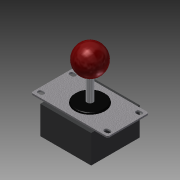
# Autodesk Inventor part: Sanwa_Joystick_JLF-TP-8YT
Saved by Autodesk Inventor 2013 (Build 170138000, 138)
## iProperties
Created: 2012-06-19
Part Number: Sanwa_Joystick_JLF-TP-8YT
Material: Generic
Document SubType Name: Sheet Metal
Designer: bbooth
Density: 1 g/cm^3
Sheet Metal Rule: Default
Author: bbooth
Autodesk Inventor part; units mm, degrees
ref_plane "YZ Plane" through (0, 0, 0) normal (1, 0, 0) x (0, 1, 0)
ref_plane "XZ Plane" through (0, 0, 0) normal (0, 1, 0) x (-1, 0, 0)
ref_plane "XY Plane" through (0, 0, 0) normal (0, 0, 1) x (1, 0, 0)
sketch "Sketch2" plane through (0, 0, 0) normal (0, 1, 0) x (-1, 0, 0)
  line L0 (-49, 26.5) -> (49, 26.5)
  line L1 (49, 26.5) -> (49, -26.5)
  line L2 (49, -26.5) -> (-49, -26.5)
  line L3 (-49, -26.5) -> (-49, 26.5)
  point P0 (0, 0)
  point P1 (0, -26.5)
  point P2 (49, 0)
  dimension "d5" = 98
  dimension "d7" = 53
  constraints: 8 end point, 2 midpoint, 2 parallel, 1 horizontal, 1 horizontal alignment, 1 perpendicular, 1 vertical alignment
  measures "d5" distance of L2.end L1.end
  measures "d7" distance between parallel lines of L0 L2
extrude "Extrusion1" add sketch "Sketch2" along normal blind 2
sketch "Sketch3" plane through (0, 2, 0) normal (0, 1, 0) x (1, 0, 0)
  line L0 (-49, -26.5) -> (49, -26.5) projected
  line L1 (49, -26.5) -> (49, 26.5) projected
  line L2 (49, 26.5) -> (-49, 26.5) projected
  line L3 (-49, 26.5) -> (-49, -26.5) projected
  arc A0 (43.75, 17.5) -> (43.75, 23) centre (43.75, 20.25) ccw
  arc A1 (41.25, 23) -> (41.25, 17.5) centre (41.25, 20.25) ccw
  line L4 (41.25, 23) -> (43.75, 23)
  line L5 (41.25, 17.5) -> (43.75, 17.5)
  arc A2 (-41.25, 17.5) -> (-41.25, 23) centre (-41.25, 20.25) ccw
  arc A3 (-43.75, 23) -> (-43.75, 17.5) centre (-43.75, 20.25) ccw
  line L6 (-43.75, 23) -> (-41.25, 23)
  line L7 (-43.75, 17.5) -> (-41.25, 17.5)
  arc A4 (43.75, -23) -> (43.75, -17.5) centre (43.75, -20.25) ccw
  arc A5 (41.25, -17.5) -> (41.25, -23) centre (41.25, -20.25) ccw
  line L8 (41.25, -17.5) -> (43.75, -17.5)
  line L9 (41.25, -23) -> (43.75, -23)
  arc A6 (-41.25, -23) -> (-41.25, -17.5) centre (-41.25, -20.25) ccw
  arc A7 (-43.75, -17.5) -> (-43.75, -23) centre (-43.75, -20.25) ccw
  line L10 (-43.75, -17.5) -> (-41.25, -17.5)
  line L11 (-43.75, -23) -> (-41.25, -23)
  point P0 (0, 0)
  dimension "d10" = 5.5
  dimension "d13" = 2.5
  dimension "d14" = 20.25
  dimension "d15" = 41.25
  dimension "d20" = 85
  dimension "d23" = 40.5
  constraints: 16 end point, 16 point on circle, 8 centre point, 2 tangent, 1 equal radius, 1 horizontal, 1 parallel, 1 perpendicular, 1 vertical, 30 other
  measures "d10" diameter of A0
  measures "d13" distance of A0.centre A1.centre
  measures "d14" vertical distance of point (0, 0) A0.centre
  measures "d15" horizontal distance of point (0, 0) A1.centre
  measures "d20" distance of A0.centre A2.centre
  measures "d23" distance of A0.centre A4.centre
extrude "Extrusion4" cut sketch "Sketch3" against normal blind 2 keep common part
sketch "Sketch4" plane through (0, 2, 0) normal (0, 1, 0) x (1, 0, 0)
  circle A0 centre (0, 0) radius 19
  dimension "d30" = 38
  constraints: 1 centre point, 1 coincident
  measures "d30" diameter of A0
extrude "Extrusion5" add sketch "Sketch4" along normal blind 2
sketch "Sketch5" plane through (0, 4, 0) normal (0, 1, 0) x (1, 0, 0)
  circle A0 centre (0, 0) radius 19 projected
  circle A1 centre (0, 0) radius 4
  dimension "d34" = 8
  constraints: 1 centre point, 1 coincident
  measures "d34" diameter of A1
extrude "Extrusion6" add sketch "Sketch5" along normal blind 46 contours A1
sketch "Sketch6" plane through (0, 0, 0) normal (0, -1, 0) x (1, 0, 0)
  line L0 (-32.5, 31) -> (32.5, 31)
  line L1 (32.5, 31) -> (32.5, -31)
  line L2 (32.5, -31) -> (-32.5, -31)
  line L3 (-32.5, -31) -> (-32.5, 31)
  point P0 (0, 0)
  point P1 (0, 31)
  point P2 (-32.5, 0)
  dimension "d39" = 65
  dimension "d42" = 62
  constraints: 8 end point, 2 midpoint, 2 parallel, 1 horizontal, 1 horizontal alignment, 1 perpendicular, 1 vertical alignment
  measures "d39" distance between parallel lines of L1 L3
  measures "d42" distance between parallel lines of L2 L0
extrude "Extrusion7" add sketch "Sketch6" along normal blind 36
sketch "Sketch7" plane through (0, 50, 0) normal (0, 1, 0) x (1, 0, 0)
  circle A0 centre (0, 0) radius 4 projected
  circle A1 centre (0, 0) radius 18
  line L0 (11.079, 14.1865) -> (-11.079, -14.1865)
  dimension "d46" = 36
  constraints: 2 end point, 2 point on circle, 1 centre point, 1 coincident, 1 midpoint
  measures "d46" diameter of A1
revolve "Revolution1" add sketch "Sketch7" angle 360 about axis through (11.079, 50, -14.1865) along (-0.6154984, 0, 0.7881381) picked at (-1.4546, 2.0706) picked at (6.9677, 11.2549) contours L0 A0 | A0 L0 A1
fillet "Fillet1" radius 2 1 edges at (49, 1, 26.5)
fillet "Fillet2" radius 2 1 edges at (49, 1, -26.5)
fillet "Fillet3" radius 2 1 edges at (-49, 1, -26.5)
fillet "Fillet4" radius 2 1 edges at (-49, 1, 26.5)
fillet "Fillet5" radius 2 1 edges at (-19, 4, 0)
equation "\"BendRadius\" = Thickness"
equation "\"BendReliefWidth\" = Thickness"
equation "\"BendReliefDepth\" = 0.5 * Thickness"
equation "\"CornerReliefSize\" = 4 * Thickness"
equation "\"MinimumRemnant\" = 2 * Thickness"
equation "\"TransitionRadius\" = BendRadius"
equation "\"JacobiRadiusSize\" = Thickness"
equation "\"GapSize\" = Thickness"
equation "\"Thickness\" = 0.5"
body "Solid1"
